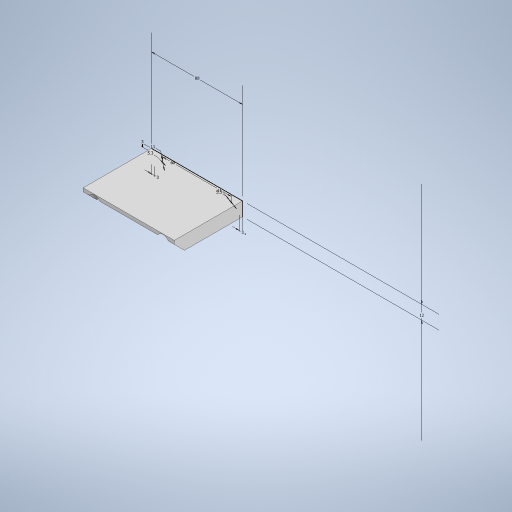
# Autodesk Inventor part: Soporte Y
Saved by Autodesk Inventor 2024 (Build 280153000, 153)
## iProperties
Created: 2024-06-03
Part Number: Soporte Y
Material: Generic
Document SubType Name: Modeling
Designer: juanp
Density: 1 g/cm^3
Appearance: Default
Author: juanp
Autodesk Inventor part; units mm, degrees
ref_plane "YZ Plane" through (0, 0, 0) normal (1, 0, 0) x (0, 1, 0)
ref_plane "XZ Plane" through (0, 0, 0) normal (0, 1, 0) x (-1, 0, 0)
ref_plane "XY Plane" through (0, 0, 0) normal (0, 0, 1) x (1, 0, 0)
sketch "Sketch1" plane through (0, 0, 0) normal (0, 0, 1) x (1, 0, 0)
  line L0 (40, -6) -> (-40, -6)
  line L1 (-40, -6) -> (-40, 6)
  line L2 (-40, 6) -> (40, 6)
  line L3 (40, 6) -> (40, -6)
  line L4 (40, -6) -> (-40, 6) construction
  line L5 (-40, -6) -> (40, 6) construction
  line L6 (-30, 0) -> (30, 0) construction
  circle A0 centre (-30, 0) radius 2.65
  circle A1 centre (30, 0) radius 2.65
  circle A2 centre (-30, 0) radius 5.5
  circle A3 centre (30, 0) radius 5.5
  line L7 (-40, 3) -> (40, 3)
  line L8 (-37, 6) -> (-37, -6)
  line L9 (37, 6) -> (37, -6)
  point P0 (0, 0)
  point P1 (-37, 3)
  point P2 (-34.6098, 3)
  point P3 (-25.3902, 3)
  point P4 (25.3902, 3)
  point P5 (34.6098, 3)
  point P6 (37, 3)
  dimension "d0" = 80
  dimension "d1" = 12
  dimension "d2" = 60
  dimension "d3" = 5.3
  dimension "d4" = 5.3
  dimension "d5" = 11
  dimension "d6" = 11
  dimension "d7" = 3
  dimension "d8" = 3
  dimension "d9" = 3
  constraints: 20 end point, 6 point on line, 4 centre point, 4 coincident, 4 perpendicular, 3 midpoint, 2 horizontal, 2 parallel
  measures "d0" distance of L1.end L2.end
  measures "d1" distance of L2.end L0.start
  measures "d2" distance of L6.start L6.end
  measures "d3" diameter of A0
  measures "d4" diameter of A1
  measures "d5" diameter of A2
  measures "d6" diameter of A3
  measures "d7" distance between parallel lines of L2 L7
  measures "d8" distance between parallel lines of L1 L8
  measures "d9" distance between parallel lines of L3 L9
extrude "Extrusion1" add sketch "Sketch1" along normal blind 3
extrude "Extrusion2" add sketch "Sketch1" along normal blind 60 contours L0 L9 L7 L3 | L7 L9 L2 L3 | L0 L1 L7 L8 | L7 A3 A2 L8 L2 L9 | L7 L1 L2 L8
chamfer "Chamfer1" distance 8.9 angle 45 2 edges at (-38.5, -6, 60) (38.5, -6, 60)
body "Solid1"
